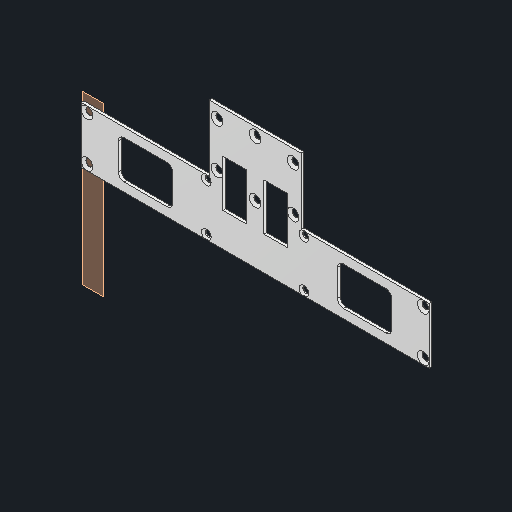
# Autodesk Inventor part: ceil
Saved by Autodesk Inventor 2023 (Build 270158000, 158)
## iProperties
Created: 2024-04-25
Part Number: ceil
Material: ABS Plastic
Document SubType Name: Modeling
Designer: szymo
Density: 1.06 g/cm^3
Appearance: Smooth - White
Mass: 7.1746 g
Surface Area: 111.011 cm^2
Volume: 6.76849 cm^3
Author: szymo
Autodesk Inventor part; units mm, degrees
ref_plane "YZ Plane" through (0, 0, 0) normal (1, 0, 0) x (0, 1, 0)
ref_plane "XZ Plane" through (0, 0, 0) normal (0, 1, 0) x (-1, 0, 0)
ref_plane "XY Plane" through (0, 0, 0) normal (0, 0, 1) x (1, 0, 0)
ref_plane "Work Plane1" through (0, 0, 0) normal (0, 0, 1) x (1, 0, 0)
ref_plane "Work Plane2" through (0, 0, 0) normal (0, 0, 1) x (1, 0, 0)
sketch "Sketch3" plane through (0, 0, 0) normal (0, 0, 1) x (1, 0, 0)
  circle A0 centre (3, -25.75) radius 2.3 projected
  circle A1 centre (3, -3) radius 2.3 projected
  circle A2 centre (3, -74.8889) radius 2.3 projected
  line L0 (0, 0) -> (6, 0) projected
  line L1 (0, -77.8889) -> (0, 0) projected
  line L2 (0, -77.8889) -> (6, -77.8889) projected
  line L3 (6, -71.8889) -> (6, -77.8889) projected
  line L4 (6, -71.8889) -> (1.6, -71.8889) projected
  line L5 (1.6, -71.8889) -> (1.6, -56.7889) projected
  line L6 (1.6, -56.7889) -> (3, -56.7889) projected
  line L7 (3, -28.75) -> (3, -56.7889) projected
  line L8 (3, -28.75) -> (6, -28.75) projected
  line L9 (6, -28.75) -> (6, -22.75) projected
  line L10 (6, -22.75) -> (3, -22.75) projected
  line L11 (3, -6) -> (3, -22.75) projected
  line L12 (3, -6) -> (6, -6) projected
  line L13 (6, -6) -> (6, 0) projected
  circle A3 centre (175, -3) radius 2.3 projected
  circle A4 centre (175, -25.75) radius 2.3 projected
  line L14 (175, -28.75) -> (175, -71.8889) projected
  line L15 (175, -6) -> (175, -22.75) projected
  line L16 (172, -71.8889) -> (172, -77.8889) projected
  line L17 (178, -77.8889) -> (172, -77.8889) projected
  line L18 (178, -77.8889) -> (178, 0) projected
  line L19 (178, 0) -> (172, 0) projected
  line L20 (172, 0) -> (172, -6) projected
  line L21 (172, -6) -> (175, -6) projected
  line L22 (175, -22.75) -> (172, -22.75) projected
  line L23 (172, -22.75) -> (172, -28.75) projected
  line L24 (172, -28.75) -> (175, -28.75) projected
  circle A5 centre (175, -74.8889) radius 2.3 projected
  circle A6 centre (89, 0.9661) radius 2.3 projected
  circle A7 centre (89, 29.5) radius 2.3 projected
  circle A8 centre (89, 15.55) radius 3.3 projected
  circle A9 centre (89, -14.375) radius 3.3 projected
  circle A10 centre (89, 41.2) radius 3.3 projected
  line L25 (93.5, -27.75) -> (84.5, -27.75) projected
  line L26 (93.5, 55) -> (93.5, -27.75) projected
  line L27 (84.5, 55) -> (93.5, 55) projected
  line L28 (84.5, -27.75) -> (84.5, 55) projected
  line L29 (105.5, -27.75) -> (111.5, -27.75) projected
  line L30 (111.5, -24.9105) -> (111.5, -27.75) projected
  arc A11 (105.5, -24.9105) -> (111.5, -24.9105) centre (108.5, -23.95) ccw projected
  line L31 (105.5, -27.75) -> (105.5, -24.9105) projected
  arc A12 (111.5, -22.9895) -> (105.5, -22.9895) centre (108.5, -23.95) ccw projected
  line L32 (111.5, -5.5855) -> (111.5, -22.9895)
  arc A13 (105.5, -5.5855) -> (111.5, -5.5855) centre (108.5, -4.625) ccw projected
  line L33 (105.5, -22.9895) -> (105.5, -5.5855) projected
  circle A14 centre (108.4846, 4.5875) radius 2.3 projected
  arc A15 (105.5, 12.8395) -> (111.5, 12.8395) centre (108.5, 13.8) ccw projected
  line L34 (105.5, -3.6645) -> (105.5, 12.8395) projected
  arc A16 (111.5, -3.6645) -> (105.5, -3.6645) centre (108.5, -4.625) ccw projected
  line L35 (111.5, 12.8395) -> (111.5, -3.6645) projected
  circle A17 centre (108.4462, 27.5) radius 2.3 projected
  arc A18 (111.5, 14.7605) -> (105.5, 14.7605) centre (108.5, 13.8) ccw projected
  line L36 (111.5, 40.6331) -> (111.5, 14.7605) projected
  arc A19 (105.5, 40.1338) -> (111.5, 40.6331) centre (108.4231, 41.3077) ccw projected
  line L37 (105.5, 14.7605) -> (105.5, 40.1338) projected
  arc A20 (111.5, 41.9823) -> (105.5, 42.4816) centre (108.4231, 41.3077) ccw projected
  line L38 (111.5, 55) -> (111.5, 41.9823) projected
  line L39 (105.5, 55) -> (111.5, 55) projected
  line L40 (105.5, 42.4816) -> (105.5, 55) projected
  line L41 (111.5, 41.9823) -> (111.5, 55) projected
  line L42 (111.5, 41.9823) -> (112.5, 41.9823) projected
  line L43 (112.5, 41.9823) -> (112.5, 55) projected
  line L44 (111.5, 55) -> (112.5, 55) projected
  line L45 (111.5, 14.7605) -> (111.5, 40.6331) projected
  line L46 (111.5, 14.7605) -> (112.5, 14.7605) projected
  line L47 (112.5, 14.7605) -> (112.5, 40.6331) projected
  line L48 (111.5, 40.6331) -> (112.5, 40.6331) projected
  line L49 (111.5, 0) -> (111.5, 12.8395) projected
  line L50 (112.5, 0) -> (112.5, 12.8395) projected
  line L51 (111.5, 12.8395) -> (112.5, 12.8395) projected
  line L52 (66.5, 14.7605) -> (66.5, 40.6331) projected
  line L53 (66.5, 40.6331) -> (65.5, 40.6331) projected
  line L54 (65.5, 14.7605) -> (65.5, 40.6331) projected
  line L55 (66.5, 14.7605) -> (65.5, 14.7605) projected
  line L56 (66.5, 41.9823) -> (66.5, 55) projected
  line L57 (66.5, 55) -> (65.5, 55) projected
  line L58 (65.5, 41.9823) -> (65.5, 55) projected
  line L59 (66.5, 41.9823) -> (65.5, 41.9823) projected
  line L60 (66.5, 0) -> (66.5, 12.8395) projected
  line L61 (66.5, 12.8395) -> (65.5, 12.8395) projected
  line L62 (65.5, 0) -> (65.5, 12.8395) projected
  arc A21 (66.5, -5.5855) -> (72.5, -5.5855) centre (69.5, -4.625) ccw projected
  line L63 (66.5, -22.9895) -> (66.5, -5.5855) projected
  arc A22 (72.5, -22.9895) -> (66.5, -22.9895) centre (69.5, -23.95) ccw projected
  line L64 (72.5, -5.5855) -> (72.5, -22.9895) projected
  line L65 (66.5, -27.75) -> (72.5, -27.75) projected
  line L66 (72.5, -24.9105) -> (72.5, -27.75) projected
  arc A23 (66.5, -24.9105) -> (72.5, -24.9105) centre (69.5, -23.95) ccw projected
  line L67 (66.5, -27.75) -> (66.5, -24.9105) projected
  circle A24 centre (69.5, 4.5875) radius 2.3 projected
  arc A25 (72.5, -3.6645) -> (66.5, -3.6645) centre (69.5, -4.625) ccw projected
  line L68 (72.5, 12.8395) -> (72.5, -3.6645) projected
  arc A26 (66.5, 12.8395) -> (72.5, 12.8395) centre (69.5, 13.8) ccw projected
  line L69 (66.5, -3.6645) -> (66.5, 12.8395) projected
  circle A27 centre (69.5, 27.5) radius 2.3 projected
  arc A28 (66.5, 40.6331) -> (72.5, 40.1338) centre (69.5769, 41.3077) ccw projected
  line L70 (66.5, 14.7605) -> (66.5, 40.6331) projected
  arc A29 (72.5, 14.7605) -> (66.5, 14.7605) centre (69.5, 13.8) ccw projected
  line L71 (72.5, 40.1338) -> (72.5, 14.7605) projected
  arc A30 (72.5, 42.4816) -> (66.5, 41.9823) centre (69.5769, 41.3077) ccw projected
  line L72 (72.5, 55) -> (72.5, 42.4816) projected
  line L73 (66.5, 55) -> (72.5, 55) projected
  line L74 (66.5, 41.9823) -> (66.5, 55) projected
  line L75 (56.8, -28.75) -> (56.8, 0) projected
  line L76 (61.8, -28.75) -> (56.8, -28.75) projected
  line L77 (61.8, 0) -> (56.8, 0) projected
  line L78 (61.8, -28.75) -> (66.3, -28.75) projected
  line L79 (66.3, 0) -> (66.3, -28.75) projected
  line L80 (61.8, 0) -> (66.3, 0) projected
  line L81 (116.2, 0) -> (111.7, 0) projected
  line L82 (111.7, 0) -> (111.7, -28.75)
  line L83 (116.2, -28.75) -> (111.7, -28.75) projected
  line L84 (121.2, -28.75) -> (121.2, 0)
  line L85 (116.2, 0) -> (121.2, 0) projected
  line L86 (116.2, -28.75) -> (121.2, -28.75) projected
  line L87 (0, 0) -> (178, 0)
  line L88 (178, 0) -> (178, -28.75)
  line L89 (178, -28.75) -> (0, -28.75)
  line L90 (0, -28.75) -> (0, 0)
  line L91 (112.5, 0) -> (65.5, 0)
  line L92 (65.5, 0) -> (65.5, 55)
  line L93 (65.5, 55) -> (112.5, 55)
  line L94 (112.5, 55) -> (112.5, 0)
  line L95 (104.5, 11.4325) -> (104.5, -10.5675) projected
  line L96 (94.5, -10.5675) -> (94.5, 11.4325) projected
  line L97 (104.5, 11.4325) -> (73.5, 11.4325)
  line L98 (73.5, 11.4325) -> (73.5, -10.5675)
  line L99 (73.5, -10.5675) -> (104.5, -10.5675)
  line L100 (104.5, -10.5675) -> (104.5, 11.4325)
  line L101 (72.5, 12.4325) -> (105.5, 12.4325)
  line L102 (105.5, 12.4325) -> (105.5, -11.5675)
  line L103 (105.5, -11.5675) -> (72.5, -11.5675)
  line L104 (72.5, -11.5675) -> (72.5, 12.4325)
  line L105 (175, -71.8889) -> (172, -71.8889) projected
  arc A31 (22.05, -4.5875) -> (19.05, -7.5875) centre (22.05, -7.5875) ccw projected
  line L106 (22.05, -4.5875) -> (43.875, -4.5875) projected
  line L107 (19.05, -21.225) -> (19.05, -7.5875) projected
  arc A32 (19.05, -21.225) -> (22.05, -24.225) centre (22.05, -21.225) ccw projected
  line L108 (43.875, -24.225) -> (22.05, -24.225) projected
  arc A33 (43.875, -24.225) -> (46.875, -21.225) centre (43.875, -21.225) ccw projected
  line L109 (46.875, -7.5875) -> (46.875, -21.225) projected
  arc A34 (46.875, -7.5875) -> (43.875, -4.5875) centre (43.875, -7.5875) ccw projected
  line L110 (134.125, -4.525) -> (155.95, -4.525) projected
  arc A35 (158.95, -7.525) -> (155.95, -4.525) centre (155.95, -7.525) ccw projected
  line L111 (158.95, -7.525) -> (158.95, -21.1625) projected
  arc A36 (155.95, -24.1625) -> (158.95, -21.1625) centre (155.95, -21.1625) ccw projected
  line L112 (155.95, -24.1625) -> (134.125, -24.1625) projected
  arc A37 (131.125, -21.1625) -> (134.125, -24.1625) centre (134.125, -21.1625) ccw projected
  line L113 (131.125, -21.1625) -> (131.125, -7.525) projected
  arc A38 (134.125, -4.525) -> (131.125, -7.525) centre (134.125, -7.525) ccw projected
  line L114 (65.5, 33.8) -> (112.5, 33.8)
  line L115 (66.5, 0) -> (65.5, 0) projected
  line L116 (111.5, 0) -> (112.5, 0) projected
  circle A39 centre (64.05, -2.25) radius 1.5 projected
  circle A40 centre (64.05, -26.5) radius 1.5 projected
  circle A41 centre (113.95, -26.5) radius 1.75 projected
  circle A42 centre (113.95, -2.25) radius 1.75 projected
  point P0 (112.5, 0)
  point P1 (65.5, 0)
  point P2 (0, -28.75)
  point P3 (172, 0)
  point P4 (93.5, 12.4325)
  point P5 (105.5, -5.5855)
  point P6 (93.5, -11.5675)
  point P7 (84.5, -11.5675)
  point P8 (72.5, -5.5855)
  point P9 (84.5, 12.4325)
  point P10 (111.5, 33.8)
  dimension "d29" = 1
  dimension "d30" = 1
  dimension "d31" = 1
  dimension "d38" = 4.6
  dimension "d39" = 4.3
  constraints: 40 end point, 8 parallel, 7 point on line, 6 perpendicular, 4 coincident, 3 horizontal, 3 other
  measures "d29" distance between parallel lines of L95 L34
  measures "d30" distance between parallel lines of L68 L98
  measures "d31" distance between parallel lines of L97 L101
  measures "d38" diameter of A7
  measures "d39" distance from line of L114 A7.centre
extrude "Extrusion2" add sketch "Sketch3" along normal blind 1.4 contours A0 | A1 | L0 L13 L12 L11 L10 L9 L8 L89 L1 | L87 L75 L89 L9 L10 L11 L12 L13 | L77 L80 L79 L78 L76 L75 | L62 L61 L60 L87 L80 | L79 L87 L69 A25 L104 A21 L63 A22 L64 L103 L28 L25 L26 L33 A12 L32 A13 L102 A16 L35 L82 L89 | L92 L55 A29 L71 L114 L28 L101 L68 A26 L61 | L82 L81 L85 L84 L86 L83 | A26 L68 L87 L60 | L54 L114 L52 L55 | L87 L68 A25 L69 | L87 L35 L51 L50 L81 | L52 L114 L71 A29 | L87 L34 A15 L35 | L35 A16 L34 L87 | L84 L87 L20 L21 L15 L22 L23 L89 | L51 A15 L34 L101 L26 L114 L37 A18 L46 L94 | L23 L22 L15 L21 L20 L19 L18 L89 L24 | L101 A8 L26 L97 L28 | L28 L114 L26 L101 A8 | L64 A22 L63 A21 | L87 A6 L26 L99 L28 | L28 L97 L26 L87 A6 | L46 L36 L114 L47 | L101 A8 | A8 L101 | L99 L26 L103 A9 L28 | L87 A6 | A6 L87 | A18 L37 L114 L36 | A13 L32 A12 L33 | L103 A9 L26 L25 L28 | L103 A9 | A9 L103 | A3 | A4 | A7 | L31 A11 L30 L29 | A14 | A17 | L67 A23 L66 L65 | A24 | A27 | A39 | A40 | A41 | A42
sketch "Sketch4" plane through (0, 0, 1.4) normal (0, 0, 1) x (1, 0, 0)
  circle A0 centre (69.5, 27.5) radius 2.3 projected
  circle A1 centre (69.5, 4.5875) radius 2.3 projected
  circle A2 centre (89, 0.9661) radius 2 projected
  circle A3 centre (89, 29.5) radius 2.3 projected
  circle A4 centre (108.4462, 27.5) radius 2.3 projected
  circle A5 centre (108.4846, 4.5875) radius 2.3 projected
  circle A6 centre (3, -25.75) radius 2.3 projected
  circle A7 centre (3, -3) radius 2.3 projected
  circle A8 centre (175, -25.75) radius 2.3 projected
  circle A9 centre (175, -3) radius 2.3 projected
  point P0 (0, 0)
  constraints: 10 coincident
hole "Hole2" at (3, -3, 1.4) at (3, -25.75, 1.4) at (175, -3, 1.4) at (175, -25.75, 1.4) at (108.4846, 4.5875, 1.4) at (89, 0.9661, 1.4) at (69.5, 4.5875, 1.4) at (69.5, 27.5, 1.4) at (89, 29.5, 1.4) at (108.4462, 27.5, 1.4) direction (0, 0, -1) diameter 3.6 end through all countersink diameter 6 countersink angle 90 clearance for "Countersunk Flat Head Screw ISO 2009/7046" size "M3" standard "ISO"
sketch "Sketch5" plane through (0, 0, 1.4) normal (0, 0, 1) x (1, 0, 0)
  circle A0 centre (64.05, -26.5) radius 1.5 projected
  circle A1 centre (113.95, -26.5) radius 1.5 projected
  circle A2 centre (64.05, -2.25) radius 1.5 projected
  circle A3 centre (113.95, -2.25) radius 1.5 projected
  point P0 (0, 0)
  constraints: 4 coincident
hole "Hole3" at (64.05, -2.25, 1.4) at (64.05, -26.5, 1.4) at (113.95, -26.5, 1.4) at (113.95, -2.25, 1.4) direction (0, 0, -1) diameter 3.1 end through all countersink diameter 5 countersink angle 90 clearance for "Countersunk Flat Head Screw ISO 2009/7046" size "M2.5" standard "ISO"
equation "\"d30\" = d29"
body "Solid2"
